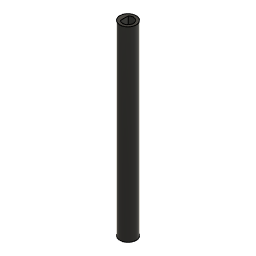
конвейер  (1) (Autodesk Fusion 360 archive; units mm, degrees)
design "трубка подлинее"
Autodesk Fusion 360 part; units mm, degrees
sketch "Sketch1" plane through (0, 0, 0) normal (0, 1, 0) x (1, 0, 0)
  circle A0 centre (0, 0) radius 3.75
  dimension "d1" = 7.5
  constraint coincident A0.centre origin
  measures "d1" diameter of A0
extrude "Extrude1" add sketch "Sketch1" along normal blind 86
sketch "Sketch2" plane through (0, 86, 0) normal (0, 1, 0) x (-1, 0, 0)
  line L0 (1.7, 0) -> (1.7, -1.833)
  line L1 (1.7, -1.833) -> (1.7, 1.833)
  arc A0 (1.7, 1.833) -> (1.7, -1.833) centre (0, 0) ccw
  dimension "d16" = 5
  dimension "d17" = 1.7
  constraint coincident A0.centre origin
  measures "d16" diameter of A0
  measures "d17" distance of A0.centre L0.start
extrude "Extrude2" cut sketch "Sketch2" against normal blind 14

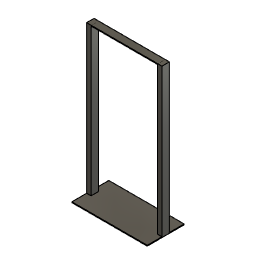
design "поддержка"
Autodesk Fusion 360 part; units mm, degrees
sketch "Sketch1" plane through (0, 0, 0) normal (0, 1, 0) x (1, 0, 0)
  line L0 (-25, 0) -> (65, 0)
  line L1 (65, 0) -> (65, 10)
  line L2 (65, 10) -> (-25, 10)
  line L3 (-25, 10) -> (-25, 0)
  line L4 (-25, 10) -> (-31, 10)
  line L5 (-31, 10) -> (-31, 0)
  line L6 (-31, 0) -> (-25, 0)
  line L7 (-25, 0) -> (-25, 10)
  line L8 (65, 10) -> (71, 10)
  line L9 (71, 10) -> (71, 0)
  line L10 (71, 0) -> (65, 0)
  line L11 (65, 0) -> (65, 10)
  line L12 (-31, 10) -> (71, 10)
  line L13 (71, 10) -> (71, 30)
  line L14 (71, 30) -> (-31, 30)
  line L15 (-31, 30) -> (-31, 10)
  line L16 (-31, 0) -> (71, 0)
  line L17 (71, 0) -> (71, -20)
  line L18 (71, -20) -> (-31, -20)
  line L19 (-31, -20) -> (-31, 0)
  dimension "d1" = 90
  dimension "d2" = 6
  dimension "d3" = 6
  dimension "d4" = 10
  dimension "d11" = 20
  dimension "d12" = 20
  constraint horizontal L0
  constraint vertical L1
  constraint horizontal L2
  constraint vertical L3
  constraint horizontal L4
  constraint vertical L5
  constraint horizontal L6
  constraint vertical L7
  constraint horizontal L8
  constraint vertical L9
  constraint horizontal L10
  constraint vertical L11
  constraint horizontal L12
  constraint vertical L13
  constraint horizontal L14
  constraint vertical L15
  constraint horizontal L16
  constraint vertical L17
  constraint horizontal L18
  constraint vertical L19
  measures "d1" distance of L0.start L0.end
  measures "d2" distance of L2.end L4.end
  measures "d3" distance of L1.end L8.end
  measures "d4" distance of L8.end L9.end
  measures "d11" distance of L4.end L14.end
  measures "d12" distance of L5.end L18.end
extrude "Extrude1" add sketch "Sketch1" along normal blind 1 contours L0 L1 L2 L3 L7 L11 L12 L16 | L3 L4 L5 L6 L7 L12 L16 | L1 L8 L9 L10 L11 L12 L16
extrude "Extrude2" add sketch "Sketch1" along normal blind 200 contours L3 L4 L5 L6 L7 L12 L16 | L1 L8 L9 L10 L11 L12 L16
sketch "Sketch2" plane through (0, 200, 0) normal (0, 1, 0) x (-1, 0, 0)
  line L0 (25, 0) -> (25, -10)
  line L1 (25, -10) -> (31, -10)
  line L2 (31, -10) -> (31, 0)
  line L3 (31, 0) -> (25, 0)
  line L4 (31, -10) -> (-65, -10)
  line L5 (-65, -10) -> (-65, 0)
  line L6 (-65, 0) -> (31, 0)
  line L7 (31, 0) -> (31, -10)
  constraint horizontal L4
  constraint vertical L5
  constraint horizontal L6
  constraint vertical L7
  constraint coincident L1.end L2.start
extrude "Extrude3" add sketch "Sketch2" 1 faces at (67, 200, -6.6667) along normal blind 1
extrude "Extrude4" add sketch "Sketch1" along normal blind 1 contours L0 L6 L10 L16 L17 L18 L19 | L2 L4 L8 L12 L13 L14 L15

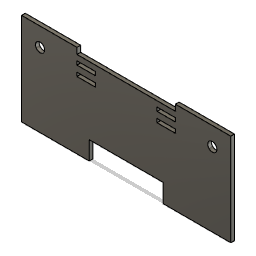
design "стенка 3"
Autodesk Fusion 360 part; units mm, degrees
sketch "Sketch1" plane through (0, 0, 0) normal (0, 1, 0) x (1, 0, 0)
sketch "Sketch2" plane through (0, 0, 0) normal (0, 0, 1) x (1, 0, 0)
  line L0 (170, 0) -> (170, 75)
  line L1 (0, 60) -> (0, 0)
  line L2 (0, 0) -> (55, 0)
  line L3 (0, 0) -> (55, 0)
  line L4 (115, 0) -> (115, 15)
  line L5 (115, 15) -> (55, 15)
  line L6 (55, 15) -> (55, 0)
  line L7 (115, 0) -> (170, 0)
  line L8 (0, 75) -> (15, 75)
  line L9 (0, 60) -> (0, 75)
  circle A0 centre (15, 60) radius 10
  circle A1 centre (155, 60) radius 10
  line L10 (15, 70) -> (155, 70)
  line L11 (155, 70) -> (155, 50)
  line L12 (155, 50) -> (15, 50)
  line L13 (15, 50) -> (15, 70)
  line L14 (0, 75) -> (45, 75)
  line L15 (125, 75) -> (125, 70)
  line L16 (125, 70) -> (45, 70)
  line L17 (45, 70) -> (45, 75)
  line L18 (170, 75) -> (125, 75)
  line L19 (45, 75) -> (15, 75)
  circle A2 centre (15, 60) radius 3.75
  circle A3 centre (155, 60) radius 3.75
  line L20 (15, 60) -> (45, 60)
  line L21 (155, 60) -> (125, 60)
  line L22 (125, 60) -> (110, 60)
  line L23 (110, 60) -> (110, 62.5)
  line L24 (110, 62.5) -> (125, 62.5)
  line L25 (125, 62.5) -> (125, 60)
  line L26 (110, 60) -> (125, 60)
  line L27 (125, 60) -> (125, 57.5)
  line L28 (125, 57.5) -> (110, 57.5)
  line L29 (110, 57.5) -> (110, 60)
  line L30 (110, 62.5) -> (125, 62.5)
  line L31 (125, 62.5) -> (125, 65.5)
  line L32 (125, 65.5) -> (110, 65.5)
  line L33 (110, 65.5) -> (110, 62.5)
  line L34 (110, 57.5) -> (125, 57.5)
  line L35 (125, 57.5) -> (125, 54.5)
  line L36 (125, 54.5) -> (110, 54.5)
  line L37 (110, 54.5) -> (110, 57.5)
  line L38 (45, 60) -> (60, 60)
  line L39 (60, 60) -> (60, 62.5)
  line L40 (60, 62.5) -> (45, 62.5)
  line L41 (45, 62.5) -> (45, 60)
  line L42 (45, 60) -> (60, 60)
  line L43 (60, 60) -> (60, 57.5)
  line L44 (60, 57.5) -> (45, 57.5)
  line L45 (45, 57.5) -> (45, 60)
  line L46 (45, 62.5) -> (60, 62.5)
  line L47 (60, 62.5) -> (60, 65.5)
  line L48 (60, 65.5) -> (45, 65.5)
  line L49 (45, 65.5) -> (45, 62.5)
  line L50 (45, 57.5) -> (60, 57.5)
  line L51 (60, 57.5) -> (60, 54.5)
  line L52 (60, 54.5) -> (45, 54.5)
  line L53 (45, 54.5) -> (45, 57.5)
  dimension "d1" = 170
  dimension "d2" = 75
  dimension "d3" = 55
  dimension "d4" = 7.5
  dimension "d5" = 7.5
  dimension "d6" = 15
  dimension "d7" = 2.5
  dimension "d8" = 2.5
  dimension "d9" = 3
  dimension "d10" = 3
  dimension "d11" = 2.5
  dimension "d12" = 15
  dimension "d13" = 30
  dimension "d14" = 2.5
  dimension "d15" = 3
  dimension "d16" = 3
  constraint vertical L0
  constraint horizontal L18
  constraint vertical L1
  constraint coincident L1.end L2.start
  constraint perpendicular L1 L3
  constraint vertical L4
  constraint horizontal L5
  constraint vertical L6
  constraint horizontal L8
  constraint vertical L9
  constraint horizontal L10
  constraint vertical L11
  constraint horizontal L12
  constraint vertical L13
  constraint coincident A1 L11.end
  constraint coincident A0 L10.start
  constraint coincident L14.end L18
  constraint vertical L15
  constraint horizontal L16
  constraint vertical L17
  constraint coincident L10 L15.end
  constraint collinear L18 L19
  constraint concentric A0 A2
  constraint concentric A1 A3
  constraint coincident A0.centre A2.centre
  constraint perpendicular L13 L20
  constraint coincident A1.centre A3.centre
  constraint perpendicular L11 L21
  constraint horizontal L22
  constraint vertical L23
  constraint horizontal L24
  constraint vertical L25
  constraint horizontal L26
  constraint vertical L27
  constraint horizontal L28
  constraint vertical L29
  constraint horizontal L30
  constraint vertical L31
  constraint horizontal L32
  constraint vertical L33
  constraint horizontal L34
  constraint vertical L35
  constraint horizontal L36
  constraint vertical L37
  constraint horizontal L38
  constraint vertical L39
  constraint horizontal L40
  constraint vertical L41
  constraint horizontal L42
  constraint vertical L43
  constraint horizontal L44
  constraint vertical L45
  constraint horizontal L46
  constraint vertical L47
  constraint horizontal L48
  constraint vertical L49
  constraint horizontal L50
  constraint vertical L51
  constraint horizontal L52
  constraint vertical L53
  measures "d1" distance of L1.end L0.start
  measures "d2" distance of L1.end L8.start
  measures "d3" distance of L1.end L2.end
  measures "d4" diameter of A2
  measures "d5" diameter of A3
  measures "d6" distance of L21.end L22.end
  measures "d7" distance of L21.end L24.end
  measures "d8" distance of L22.end L28.end
  measures "d9" distance of L23.end L32.end
  measures "d10" distance of L28.end L36.end
  measures "d11" distance of L20.end L40.end
  measures "d12" distance of L39.end L40.end
  measures "d13" distance of A0.centre L20.end
  measures "d14" distance of L20.end L44.end
  measures "d15" distance of L40.end L48.end
  measures "d16" distance of L44.end L52.end
extrude "Extrude1" add sketch "Sketch2" along normal blind 3 contours L0 L1 L2 L3 L4 L5 L6 L7 L8 L9 A0 A1 L10 L12 L14 L15 L17 L18 L19 | A0 A1 L10 L12 L16 | A1 L11 A3 L21 | A1 L11 A3 | A0 L13 A2 | A0 L13 A2 L20 | A1 L11 A3 L21 | A0 L13 A2 L20 | L22 L26 L27 L28 L29 L34 | L22 L23 L24 L25 L26 L30 | L38 L39 L40 L41 L42 L46 | L38 L42 L43 L44 L45 L50

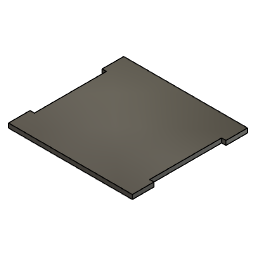
design "поддержка ооо"
Autodesk Fusion 360 part; units mm, degrees
sketch "Sketch1" plane through (0, 0, 0) normal (0, 1, 0) x (1, 0, 0)
  line L0 (0, 0) -> (80, 0)
  line L1 (80, 15) -> (80, 65)
  line L2 (80, 80) -> (0, 80)
  line L3 (0, 65) -> (0, 15)
  line L4 (0, 80) -> (-3, 80)
  line L5 (-3, 80) -> (-3, 65)
  line L6 (-3, 65) -> (0, 65)
  line L7 (0, 0) -> (-3, 0)
  line L8 (-3, 0) -> (-3, 15)
  line L9 (-3, 15) -> (0, 15)
  line L10 (80, 80) -> (83, 80)
  line L11 (83, 80) -> (83, 65)
  line L12 (83, 65) -> (80, 65)
  line L13 (80, 0) -> (83, 0)
  line L14 (83, 0) -> (83, 15)
  line L15 (83, 15) -> (80, 15)
  dimension "d15" = 80
  dimension "d16" = 80
  dimension "d17" = 3
  dimension "d18" = 3
  dimension "d19" = 3
  dimension "d20" = 3
  dimension "d21" = 15
  dimension "d22" = 15
  dimension "d23" = 15
  dimension "d24" = 15
  constraint horizontal L0
  constraint vertical L1
  constraint horizontal L2
  constraint vertical L3
  constraint coincident L0.start L7.start
  constraint horizontal L4
  constraint vertical L5
  constraint horizontal L6
  constraint horizontal L7
  constraint vertical L8
  constraint horizontal L9
  constraint horizontal L10
  constraint vertical L11
  constraint horizontal L12
  constraint horizontal L13
  constraint vertical L14
  constraint horizontal L15
  measures "d15" distance of L0.start L0.end
  measures "d16" distance of L0.start L2.end
  measures "d17" distance of L2.end L4.end
  measures "d18" distance of L0.start L7.end
  measures "d19" distance of L2.start L10.end
  measures "d20" distance of L0.end L13.end
  measures "d21" distance of L10.end L11.end
  measures "d22" distance of L4.end L5.end
  measures "d23" distance of L7.end L8.end
  measures "d24" distance of L13.end L14.end
extrude "Extrude1" add sketch "Sketch1" along normal blind 3

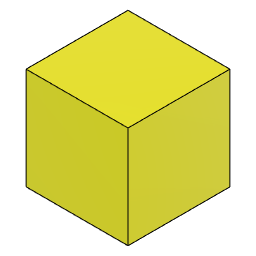
design "кубик, желтый как снег зимой"
Autodesk Fusion 360 part; units mm, degrees
sketch "Sketch1" plane through (0, 0, 0) normal (0, 1, 0) x (1, 0, 0)
  line L0 (0, 0) -> (25, 0)
  line L1 (25, 0) -> (25, 25)
  line L2 (25, 25) -> (0, 25)
  line L3 (0, 25) -> (0, 0)
  constraint horizontal L0
  constraint vertical L1
  constraint horizontal L2
  constraint vertical L3
  constraint coincident L0.start L3.end
extrude "Extrude1" add sketch "Sketch1" along normal blind 25

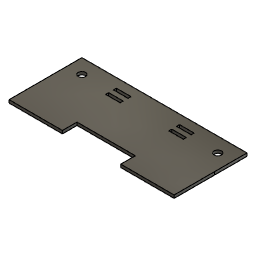
design "основа 2"
Autodesk Fusion 360 part; units mm, degrees
sketch "Sketch1" plane through (0, 0, 0) normal (0, 1, 0) x (1, 0, 0)
  circle A0 centre (25.0011, 78.3582) radius 11
  circle A1 centre (165.0011, 78.3582) radius 11
  line L0 (25.0011, 78.3582) -> (165.0011, 78.3582)
  line L1 (165.0011, 78.3582) -> (165.0011, 89.3582)
  line L2 (165.0011, 89.3582) -> (25.0011, 89.3582)
  line L3 (25.0011, 89.3582) -> (25.0011, 78.3582)
  line L4 (25.0011, 78.3582) -> (165.0011, 78.3582)
  line L5 (165.0011, 78.3582) -> (165.0011, 67.3582)
  line L6 (165.0011, 67.3582) -> (25.0011, 67.3582)
  line L7 (25.0011, 67.3582) -> (25.0011, 78.3582)
  line L8 (25.0011, 78.3582) -> (55.0011, 78.3582)
  line L9 (55.0011, 78.3582) -> (55.0011, 83.8582)
  line L10 (55.0011, 78.3582) -> (55.0011, 72.8582)
  line L11 (55.0011, 83.8582) -> (70, 83.8582)
  line L12 (70, 83.8582) -> (70, 80.8582)
  line L13 (70, 80.8582) -> (55.0011, 80.8582)
  line L14 (55.0011, 72.8582) -> (70, 72.8582)
  line L15 (70, 72.8582) -> (70, 75.8582)
  line L16 (70, 75.8582) -> (55.0011, 75.8582)
  line L17 (165.0011, 78.3582) -> (135.0011, 78.3582)
  line L18 (135.0011, 78.3582) -> (135.0011, 83.8582)
  line L19 (135.0011, 78.3582) -> (135.0011, 72.8582)
  line L20 (135.0011, 83.8582) -> (120.0011, 83.8582)
  line L21 (120.0011, 83.8582) -> (120.0011, 80.8582)
  line L22 (120.0011, 80.8582) -> (135.0011, 80.8582)
  line L23 (135.0011, 72.8582) -> (120, 72.8582)
  line L24 (120, 72.8582) -> (120, 75.8582)
  line L25 (120, 75.8582) -> (135.0011, 75.8582)
  line L26 (10.0011, 93.3582) -> (180, 93.3582)
  line L27 (180, 93.3582) -> (180, 60)
  line L28 (180, 60) -> (10.0011, 60)
  line L29 (10.0011, 60) -> (10.0011, 93.3582)
  line L30 (10.0011, 60) -> (180.0011, 60)
  line L31 (180.0011, 60) -> (180.0011, 18.3582)
  line L32 (10.0011, 18.3582) -> (10.0011, 60)
  line L33 (10.0011, 18.3582) -> (95.0011, 18.3582)
  line L34 (125.0011, 18.3582) -> (125.0011, 33.3582)
  line L35 (125.0011, 33.3582) -> (95, 33.3582)
  line L36 (95, 33.3582) -> (64.9674, 33.3582)
  line L37 (64.9674, 33.3582) -> (64.9674, 18.3582)
  line L38 (64.9674, 18.3582) -> (95, 18.3582)
  line L39 (180.0011, 18.3582) -> (125.0011, 18.3582)
  line L40 (64.9674, 18.3582) -> (10.0011, 18.3582)
  circle A2 centre (25.0011, 78.3582) radius 3.75
  circle A3 centre (165.0011, 78.3582) radius 3.75
  dimension "d64" = 22
  dimension "d65" = 22
  dimension "d66" = 140
  dimension "d67" = 11
  dimension "d68" = 140
  dimension "d69" = 11
  dimension "d70" = 30
  dimension "d71" = 5.5
  dimension "d72" = 5.5
  dimension "d73" = 3
  dimension "d74" = 3
  dimension "d75" = 30
  dimension "d76" = 5.5
  dimension "d77" = 5.5
  dimension "d78" = 15
  dimension "d79" = 3
  dimension "d80" = 3
  dimension "d81" = 170
  dimension "d82" = 85
  dimension "d83" = 7.5
  dimension "d84" = 7.5
  dimension "d85" = 75
  dimension "d86" = 15
  dimension "d87" = 55
  dimension "d88" = 15
  dimension "d89" = 15
  constraint horizontal L0
  constraint vertical L1
  constraint horizontal L2
  constraint vertical L3
  constraint coincident A0.centre L0.start
  constraint coincident A1.centre L0.end
  constraint horizontal L4
  constraint vertical L5
  constraint horizontal L6
  constraint vertical L7
  constraint perpendicular L3 L8
  constraint perpendicular L8 L9
  constraint perpendicular L8 L10
  constraint perpendicular L9 L11
  constraint perpendicular L11 L12
  constraint coincident L9 L13.end
  constraint perpendicular L9 L13
  constraint perpendicular L10 L14
  constraint perpendicular L14 L15
  constraint coincident L10 L16.end
  constraint perpendicular L10 L16
  constraint perpendicular L1 L17
  constraint perpendicular L4 L18
  constraint perpendicular L17 L19
  constraint perpendicular L18 L20
  constraint perpendicular L20 L21
  constraint coincident L18 L22.end
  constraint perpendicular L18 L22
  constraint perpendicular L19 L23
  constraint perpendicular L23 L24
  constraint coincident L19 L25.end
  constraint perpendicular L19 L25
  constraint horizontal L26
  constraint vertical L27
  constraint horizontal L28
  constraint vertical L29
  constraint horizontal L30
  constraint vertical L31
  constraint horizontal L39
  constraint vertical L32
  constraint perpendicular L32 L33
  constraint vertical L34
  constraint horizontal L35
  constraint horizontal L36
  constraint vertical L37
  constraint horizontal L38
  constraint coincident L33 L37.end
  constraint collinear L39 L40
  constraint concentric A0 A2
  measures "d64" diameter of A0
  measures "d65" diameter of A1
  measures "d66" distance of A0.centre A1.centre
  measures "d67" distance of A0.centre L2.end
  measures "d68" distance of A0.centre A1.centre
  measures "d69" distance of A0.centre L6.end
  measures "d70" distance of A0.centre L8.end
  measures "d71" distance of L8.end L9.end
  measures "d72" distance of L8.end L10.end
  measures "d73" distance of L11.end L12.end
  measures "d74" distance of L14.end L15.end
  measures "d75" distance of A1.centre L17.end
  measures "d76" distance of L17.end L18.end
  measures "d77" distance of L17.end L19.end
  measures "d78" distance of L18.end L20.end
  measures "d79" distance of L20.end L21.end
  measures "d80" distance of L23.end L24.end
  measures "d81" distance of L31.end L32.start
  measures "d82" distance of L32.start L33.end
  measures "d83" diameter of A2
  measures "d84" diameter of A3
  measures "d85" distance of L26 L33
  measures "d86" distance of L36.end L37.end
  measures "d87" distance of L31.end L34.start
  measures "d88" distance of L29 A0.centre
  measures "d89" distance of L26 A0.centre
extrude "Extrude1" add sketch "Sketch1" along normal blind 3 contours A0 L0 L3 L4 L8 A2 | A0 A1 L0 L4 L6 L8 L17 | A0 L0 L4 L7 L8 A2 | A0 A1 L0 L2 L4 L8 L17 | A0 L3 L7 A2 | A1 L0 L1 L4 L17 A3 | A1 L1 L5 A3 | A1 L0 L4 L5 L17 A3 | L26 L27 L28 L29 L30 | L28 L30 L31 L32 L33 L34 L35 L36 L37 L39 L40
sketch "Sketch2" plane through (0, 3, 0) normal (0, 1, 0) x (-1, 0, 0)
  circle A0 centre (-25.0011, -78.3582) radius 3.75
  circle A1 centre (-165.0011, -78.3582) radius 3.75
  line L0 (-135.0011, -75.8582) -> (-135.0011, -72.8582)
  line L1 (-135.0011, -72.8582) -> (-120, -72.8582)
  line L2 (-120, -72.8582) -> (-120, -75.8582)
  line L3 (-120, -75.8582) -> (-135.0011, -75.8582)
  line L4 (-135.0011, -80.8582) -> (-120.0011, -80.8582)
  line L5 (-120.0011, -80.8582) -> (-120.0011, -83.8582)
  line L6 (-120.0011, -83.8582) -> (-135.0011, -83.8582)
  line L7 (-135.0011, -83.8582) -> (-135.0011, -80.8582)
  line L8 (-55.0011, -75.8582) -> (-70, -75.8582)
  line L9 (-70, -75.8582) -> (-70, -72.8582)
  line L10 (-70, -72.8582) -> (-55.0011, -72.8582)
  line L11 (-55.0011, -72.8582) -> (-55.0011, -75.8582)
  line L12 (-55.0011, -80.8582) -> (-55.0011, -83.8582)
  line L13 (-55.0011, -83.8582) -> (-70, -83.8582)
  line L14 (-70, -83.8582) -> (-70, -80.8582)
  line L15 (-70, -80.8582) -> (-55.0011, -80.8582)
  line L16 (-64.9674, -18.3582) -> (-64.9674, -33.3582)
  line L17 (-64.9674, -33.3582) -> (-125.0011, -33.3582)
  line L18 (-125.0011, -33.3582) -> (-125.0011, -18.3582)
  line L19 (-125.0011, -18.3582) -> (-180.0011, -18.3582)
  line L20 (-180.0011, -18.3582) -> (-180.0011, -60)
  line L21 (-180.0011, -60) -> (-180, -60)
  line L22 (-180, -60) -> (-180, -93.3582)
  line L23 (-180, -93.3582) -> (-10.0011, -93.3582)
  line L24 (-10.0011, -93.3582) -> (-10.0011, -18.3582)
  line L25 (-10.0011, -18.3582) -> (-64.9674, -18.3582)
  line L26 (-23.3011, -78.3582) -> (-23.3011, -80.1912)
  line L27 (-23.3011, -80.1912) -> (-23.3011, -76.5252)
  arc A2 (-23.3011, -76.5252) -> (-23.3011, -80.1912) centre (-25.0011, -78.3582) ccw
  line L28 (-23.3011, -80.1912) -> (-23.3011, -75.0157)
  line L29 (-25.0011, -78.3582) -> (-23.5011, -78.3582)
  line L30 (-25.0011, -78.3582) -> (-26.5011, -78.3582)
  line L31 (-23.5011, -78.3582) -> (-23.5011, -57.3582)
  line L32 (-23.5011, -57.3582) -> (-26.5011, -57.3582)
  dimension "d90" = 5
  dimension "d91" = 1.7
  dimension "d93" = 1.5
  dimension "d94" = 1.5
  dimension "d95" = 3
  constraint concentric A0 A2
  constraint parallel L27 L28
  constraint coincident A0.centre A2.centre
  constraint perpendicular L26 L29
  constraint parallel L29 L30
  constraint perpendicular L23 L31
  constraint perpendicular L28 L32
  constraint coincident A0 L28.end
  measures "d90" diameter of A2
  measures "d91" distance of A0.centre L26.start
  measures "d93" distance of A0.centre L29.end
  measures "d94" distance of A0.centre L30.end
  measures "d95" distance of L31.end L32.end

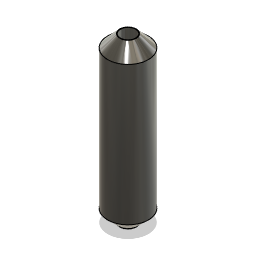
design "барабан"
Autodesk Fusion 360 part; units mm, degrees
sketch "Sketch1" plane through (0, 0, 0) normal (0, 1, 0) x (1, 0, 0)
  circle A0 centre (0, 0) radius 10
  circle A1 centre (0, 0) radius 3.75
  dimension "d4" = 20
  dimension "d8" = 7.5
  constraint coincident A0.centre A1.centre
  measures "d4" diameter of A0
  measures "d8" diameter of A1
extrude "Extrude1" add sketch "Sketch1" along normal blind 80
chamfer "Chamfer1" distance 6 angle 45 2 edges at (-9.3233, 80, 3.6162) (-9.3233, 0, 3.6162)

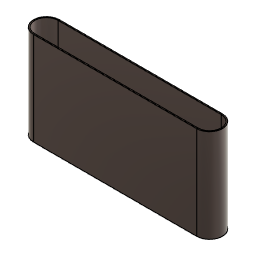
design "тяговый элемент"
Autodesk Fusion 360 part; units mm, degrees
sketch "Sketch1" plane through (0, 0, 0) normal (0, 1, 0) x (1, 0, 0)
  line L0 (140, 10) -> (0, 10)
  line L1 (0, -10) -> (140, -10)
  line L2 (0, 11) -> (140, 11)
  line L3 (0, -11) -> (140, -11)
  arc A0 (0, 11) -> (0, -11) centre (0, 0) ccw
  arc A1 (0, 10) -> (0, -10) centre (0, 0) ccw
  arc A2 (140, -10) -> (140, 10) centre (140, 0) ccw
  arc A3 (140, -11) -> (140, 11) centre (140, 0) ccw
  dimension "d8" = 140
  dimension "d9" = 10
  dimension "d10" = 22
  dimension "d11" = 22
  constraint horizontal L0
  constraint coincident A0.centre A1.centre
  constraint concentric A2 A3
  constraint tangent L1 A2
  constraint horizontal L1
  constraint tangent L2 A3
  constraint parallel L0 L2
  constraint tangent L3 A3
  constraint parallel L2 L3
  measures "d8" distance of A0.centre A2.centre
  measures "d9" distance of A0.centre L0.end
  measures "d10" diameter of A3
  measures "d11" diameter of A0
extrude "Extrude1" add sketch "Sketch1" along normal blind 80

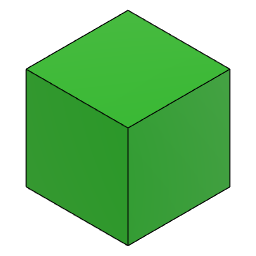
design "кубик зелененький)"
Autodesk Fusion 360 part; units mm, degrees
sketch "Sketch1" plane through (0, 0, 0) normal (0, 1, 0) x (1, 0, 0)
  line L0 (0, 0) -> (25, 0)
  line L1 (25, 0) -> (25, 25)
  line L2 (25, 25) -> (0, 25)
  line L3 (0, 25) -> (0, 0)
  constraint horizontal L0
  constraint vertical L1
  constraint horizontal L2
  constraint vertical L3
  constraint coincident L0.start L3.end
extrude "Extrude1" add sketch "Sketch1" along normal blind 25

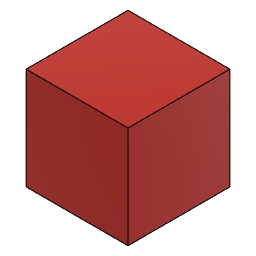
design "кубик"
Autodesk Fusion 360 part; units mm, degrees
sketch "Sketch1" plane through (0, 0, 0) normal (0, 1, 0) x (1, 0, 0)
  line L0 (0, 0) -> (25, 0)
  line L1 (25, 0) -> (25, 25)
  line L2 (25, 25) -> (0, 25)
  line L3 (0, 25) -> (0, 0)
  constraint horizontal L0
  constraint vertical L1
  constraint horizontal L2
  constraint vertical L3
  constraint coincident L0.start L3.end
extrude "Extrude1" add sketch "Sketch1" along normal blind 25

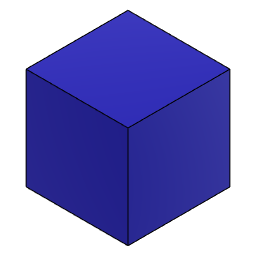
design "кубик синий"
Autodesk Fusion 360 part; units mm, degrees
sketch "Sketch1" plane through (0, 0, 0) normal (0, 1, 0) x (1, 0, 0)
  line L0 (0, 0) -> (25, 0)
  line L1 (25, 0) -> (25, 25)
  line L2 (25, 25) -> (0, 25)
  line L3 (0, 25) -> (0, 0)
  constraint horizontal L0
  constraint vertical L1
  constraint horizontal L2
  constraint vertical L3
  constraint coincident L0.start L3.end
extrude "Extrude1" add sketch "Sketch1" along normal blind 25

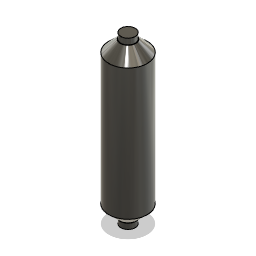
design "барабан"
Autodesk Fusion 360 part; units mm, degrees
sketch "Sketch1" plane through (0, 0, 0) normal (0, 1, 0) x (1, 0, 0)
  circle A0 centre (0, 0) radius 3.75
  circle A1 centre (0, 0) radius 10
  dimension "d1" = 7.5
  dimension "d2" = 20
  constraint coincident A0.centre A1.centre
  measures "d1" diameter of A0
  measures "d2" diameter of A1
extrude "Extrude1" add sketch "Sketch1" along normal blind 83 and the other way blind 3 contours A0
extrude "Extrude2" add sketch "Sketch1" along normal blind 80
chamfer "Chamfer1" distance 6 angle 45 2 edges at (-9.3233, 80, 3.6162) (-9.3233, 0, 3.6162)
